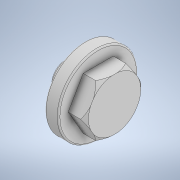
# Autodesk Inventor part: Слив_масла
Saved by Autodesk Inventor 2021 (Build 250183000, 183)
## iProperties
Created: 2023-04-23
Part Number: Слив_масла
Material: Типовые
Document SubType Name: Modeling
Designer: gdevc
Density: 1 g/cm^3
Appearance: По умолчанию
Author: gdevc
Autodesk Inventor part; units mm, degrees
ref_plane "YZ Plane" through (0, 0, 0) normal (1, 0, 0) x (0, 1, 0)
ref_plane "XZ Plane" through (0, 0, 0) normal (0, 1, 0) x (-1, 0, 0)
ref_plane "XY Plane" through (0, 0, 0) normal (0, 0, 1) x (1, 0, 0)
sketch "Эскиз1" plane through (0, 0, 0) normal (0, 0, 1) x (1, 0, 0)
  line L0 (0, 0) -> (21.2967, 0)
  line L1 (0, 0) -> (0, 6)
  line L2 (0, 6) -> (6, 6)
  line L3 (6, 6) -> (6, 5)
  line L4 (6, 5) -> (7, 5)
  line L5 (7, 5) -> (7, 14.5)
  line L6 (7, 14.5) -> (12, 14.5)
  line L7 (12, 14.5) -> (12, 0)
  dimension "d0" = 12
  dimension "d1" = 10
  dimension "d2" = 29
  dimension "d3" = 1
  dimension "d4" = 6
  dimension "d5" = 5
  constraints: 16 end point, 4 perpendicular, 3 vertical, 1 horizontal, 1 point on line
  measures "d0" diameter of L2 L0
  measures "d1" diameter of L4 L0
  measures "d2" diameter of L6 L0
  measures "d3" distance between parallel lines of L5 L3
  measures "d4" distance between parallel lines of L1 L3
  measures "d5" distance between parallel lines of L5 L7
revolve "Вращение1" add sketch "Эскиз1" angle 360 about axis through (0, 0, 0) along (1, 0, 0)
chamfer "Фаска1" distance 1 angle 45 1 edges at (0, -6, 0)
fillet "Сопряжение1" radius 0.5 2 edges at (7, -14.5, 0) (12, -14.5, 0)
sketch "Эскиз2" plane through (12, 0, 0) normal (1, 0, 0) x (0, 0, -1)
  line L0 (5.4848, 9.5) -> (10.9697, 0)
  line L1 (10.9697, 0) -> (5.4848, -9.5)
  line L2 (5.4848, -9.5) -> (-5.4848, -9.5)
  line L3 (-5.4848, -9.5) -> (-10.9697, 0)
  line L4 (-10.9697, 0) -> (-5.4848, 9.5)
  line L5 (-5.4848, 9.5) -> (5.4848, 9.5)
  point P0 (0, 0)
  point P1 (0, 0)
  dimension "d11" = 19
  constraints: 12 end point, 1 coincident, 13 other
  measures "d11" distance between parallel lines of L2 L5
extrude "Выдавливание1" add sketch "Эскиз2" along normal blind 6
sketch "Эскиз3" plane through (0, 0, 0) normal (0, 1, 0) x (-1, 0, 0)
  line L0 (-12, 10.9697) -> (-18, 10.9697) projected
  line L1 (-16.5858, 10.9697) -> (-18, 9.5554)
  line L2 (-18, 5.4848) -> (-18, 10.9697) projected
  line L3 (3.6, 0) -> (-21.6, 0) projected
  point P0 (0, 0)
  dimension "d14" = 2
  dimension "d15" = 45
  constraints: 2 end point, 2 point on line
  measures "d14" distance of L1.start L1.end
  measures "d15" angle of L2 L1
revolve "Вращение2" cut sketch "Эскиз3" angle 360 about axis through (-10, 0, 0) along (1, 0, 0)
